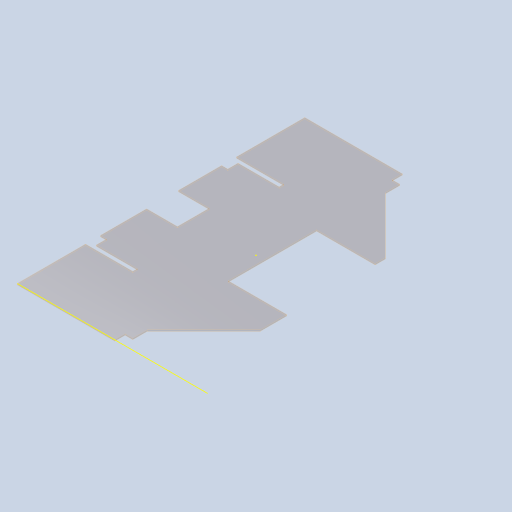
# Autodesk Inventor part: DB1-015
Saved by Autodesk Inventor 2023.4 (Build 274418000, 418)
## iProperties
Created: 2025-02-19
Part Number: DB1-015
Material: Polycarbonate, Smoke
Document SubType Name: Sheet Metal
Designer: AIM
Density: 1.2 g/cm^3
Sheet Metal Rule: Default
Appearance: Polycarbonate - Smoked
Author: AIM
Autodesk Inventor part; units mm, degrees
ref_plane "YZ Plane" through (0, 0, 0) normal (1, 0, 0) x (0, 1, 0)
ref_plane "XZ Plane" through (0, 0, 0) normal (0, 1, 0) x (-1, 0, 0)
ref_plane "XY Plane" through (0, 0, 0) normal (0, 0, 1) x (1, 0, 0)
sketch "Sketch1" plane through (0, 0, 0) normal (0, 1, 0) x (-1, 0, 0)
  line L0 (234.95, 355.6) -> (-234.95, 355.6)
  line L1 (-234.95, 355.6) -> (-234.95, -355.6)
  line L2 (-234.95, -355.6) -> (234.95, -355.6)
  line L3 (234.95, -355.6) -> (234.95, 355.6)
  line L4 (234.95, 355.6) -> (-234.95, -355.6) construction
  line L5 (-234.95, 355.6) -> (234.95, -355.6) construction
  point P0 (0, 0)
  dimension "d0" = 469.9
  dimension "d1" = 711.2
  measures "d0" distance of L2.end L1.end
  measures "d1" distance of L1.end L0.end
extrude "Plate1" add sketch "Sketch1" along normal blind 3.048
sketch "Sketch3" plane through (0, 3.048, 0) normal (0, 1, 0) x (1, 0, 0)
  line L0 (234.95, -355.6) -> (-234.95, -355.6) projected
  point P0 (0, 0)
sketch "Sketch4" plane through (0, 0, 0) normal (0, -1, 0) x (1, 0, 0)
  line L0 (-234.95, 355.6) -> (234.95, 355.6) projected
  line L1 (-234.95, -355.6) -> (-234.95, 355.6) projected
  line L2 (234.95, -355.6) -> (-234.95, -355.6) projected
  line L3 (234.95, 355.6) -> (234.95, -355.6) projected
  line L4 (-234.95, 355.6) -> (234.95, 355.6) projected
  line L5 (25.4, 355.6) -> (25.4, 294.64)
  line L6 (165.1, 101.6) -> (234.95, 101.6)
  line L7 (234.95, 355.6) -> (234.95, -355.6) projected
  line L8 (25.4, 294.64) -> (165.1, 154.94)
  line L9 (25.4, 294.64) -> (222.9656, 294.64) construction
  line L10 (165.1, 154.94) -> (165.1, 101.6)
  line L11 (234.95, 0) -> (-234.95, 0)
  line L12 (-234.95, -355.6) -> (-234.95, 355.6) projected
  line L13 (25.4, -355.6) -> (25.4, -294.64)
  line L14 (165.1, -127) -> (234.95, -127)
  line L15 (25.4, -294.64) -> (165.1, -154.94)
  line L16 (25.4, -294.64) -> (222.9656, -294.64) construction
  line L17 (165.1, -154.94) -> (165.1, -127)
  line L18 (-234.95, 184.15) -> (-120.65, 184.15)
  line L19 (-120.65, 184.15) -> (-120.65, 177.8)
  line L20 (-120.65, 177.8) -> (-222.25, 177.8)
  line L21 (-222.25, 177.8) -> (-222.25, 152.4)
  line L22 (-222.25, 152.4) -> (-234.95, 152.4)
  line L23 (-234.95, 149.86) -> (-219.71, 149.86)
  line L24 (-219.71, 149.86) -> (-219.71, 175.26)
  line L25 (-219.71, 175.26) -> (-118.11, 175.26)
  line L26 (-118.11, 175.26) -> (-118.11, 186.69)
  line L27 (-118.11, 186.69) -> (-234.95, 186.69)
  line L28 (165.1, -129.54) -> (20.32, -129.54)
  line L29 (20.32, -129.54) -> (20.32, 88.9)
  line L30 (20.32, 88.9) -> (165.1, 88.9)
  line L31 (165.1, 101.6) -> (165.1, 88.9)
  line L32 (-234.95, -184.15) -> (-120.65, -184.15)
  line L33 (-120.65, -184.15) -> (-120.65, -177.8)
  line L34 (-120.65, -177.8) -> (-222.25, -177.8)
  line L35 (-222.25, -177.8) -> (-222.25, -152.4)
  line L36 (-222.25, -152.4) -> (-234.95, -152.4)
  line L37 (-234.95, -149.86) -> (-219.71, -149.86)
  line L38 (-219.71, -149.86) -> (-219.71, -175.26)
  line L39 (-219.71, -175.26) -> (-118.11, -175.26)
  line L40 (-118.11, -175.26) -> (-118.11, -186.69)
  line L41 (-118.11, -186.69) -> (-234.95, -186.69)
  line L42 (-158.75, 35.56) -> (-158.75, -43.18)
  line L43 (-158.75, -43.18) -> (-234.95, -43.18)
  line L44 (-158.75, 35.56) -> (-234.95, 35.56)
  line L45 (25.4, 330.2) -> (6.35, 330.2)
  line L46 (6.35, 330.2) -> (6.35, 355.6)
  line L47 (25.4, -330.2) -> (6.35, -330.2)
  line L48 (6.35, -330.2) -> (6.35, -355.6)
  line L49 (234.95, -355.6) -> (-234.95, -355.6) projected
  point P0 (0, 0)
  dimension "d3" = 209.55
  dimension "d4" = 254
  dimension "d5" = 45
  dimension "d6" = 60.96
  dimension "d9" = 69.85
  dimension "d12" = 45
  dimension "d13" = 209.55
  dimension "d14" = 228.6
  dimension "d15" = 69.85
  dimension "d16" = 60.96
  dimension "d17" = 171.45
  dimension "d18" = 114.3
  dimension "d19" = 6.35
  dimension "d21" = 101.6
  dimension "d22" = 25.4
  dimension "d23" = 2.54
  dimension "d26" = 144.78
  dimension "d31" = 12.7
  dimension "d32" = 114.3
  dimension "d33" = 171.45
  dimension "d34" = 6.35
  dimension "d35" = 101.6
  dimension "d36" = 25.4
  dimension "d37" = 2.54
  dimension "d38" = 76.2
  dimension "d39" = 35.56
  dimension "d40" = 43.18
  dimension "d41" = 2.54
  dimension "d42" = 25.4
  dimension "d43" = 19.05
  dimension "d44" = 25.4
  dimension "d45" = 19.05
  constraints: 84 end point, 14 horizontal, 11 point on line, 8 vertical, 4 perpendicular, 2 midpoint, 1 equal length, 1 vertical alignment, 19 other
  measures "d3" distance between parallel lines of L3 L5
  measures "d4" distance between parallel lines of L0 L6
  measures "d5" angle of L8 L9
  measures "d6" distance from line of L5.end L0
  measures "d9" distance between parallel lines of L3 L10
  measures "d12" angle of L15 L16
  measures "d13" distance between parallel lines of L3 L13
  measures "d14" distance between parallel lines of L2 L14
  measures "d15" distance between parallel lines of L3 L17
  measures "d16" distance from line of L13.end L2
  measures "d17" distance between parallel lines of L0 L18
  measures "d18" distance of L18.start L18.end
  measures "d19" distance of L18.end L19.end
  measures "d21" distance of L19.end L20.end
  measures "d22" distance of L20.end L21.end
  measures "d23" distance between parallel lines of L20 L25
  measures "d26" distance of L28.start L28.end
  measures "d31" distance of L6.start L30.end
  measures "d32" distance of L32.start L32.end
  measures "d33" distance between parallel lines of L2 L32
  measures "d34" distance of L32.end L33.end
  measures "d35" distance of L33.end L34.end
  measures "d36" distance of L34.end L35.end
  measures "d37" distance between parallel lines of L34 L39
  measures "d38" distance between parallel lines of L1 L42
  measures "d39" distance from line of point (-234.95, 0) L44
  measures "d40" distance from line of point (-234.95, 0) L43
  measures "d41" distance of L14.start L28.start
  measures "d42" distance of L45.end L46.end
  measures "d43" distance of L45.start L45.end
  measures "d44" distance of L47.end L48.end
  measures "d45" distance of L47.start L47.end
extrude "Cut1" cut sketch "Sketch4" against normal blind 3.048 contours L27 L26 L25 L24 L23 L1 L22 L21 L20 L19 L18 | L0 L3 L6 L10 L8 L5 | L18 L19 L20 L21 L22 L1 | L3 L11 L29 L30 L31 L6 | L3 L14 L17 L28 L29 L11 | L44 L42 L11 L1 | L3 L2 L13 L15 L17 L14 | L11 L42 L43 L1 | L37 L38 L39 L40 L41 L1 L32 L33 L34 L35 L36 | L36 L35 L34 L33 L32 L1
sketch "Sketch5" plane through (0, 0, 0) normal (0, -1, 0) x (1, 0, 0)
  line L0 (25.4, 355.6) -> (25.4, 294.64) projected
  line L1 (25.4, 294.64) -> (165.1, 154.94) projected
  line L2 (165.1, 154.94) -> (165.1, 88.9) projected
  line L3 (165.1, 88.9) -> (20.32, 88.9) projected
  line L4 (20.32, 88.9) -> (20.32, -129.54) projected
  line L5 (20.32, -129.54) -> (165.1, -129.54) projected
  line L6 (165.1, -129.54) -> (165.1, -154.94) projected
  line L7 (165.1, -154.94) -> (25.4, -294.64) projected
  line L8 (25.4, -294.64) -> (25.4, -355.6) projected
  line L9 (25.4, -355.6) -> (-234.95, -355.6) projected
  line L10 (-234.95, -355.6) -> (-234.95, -186.69) projected
  line L11 (-234.95, -186.69) -> (-118.11, -186.69) projected
  line L12 (-118.11, -186.69) -> (-118.11, -175.26) projected
  line L13 (-118.11, -175.26) -> (-219.71, -175.26) projected
  line L14 (-219.71, -175.26) -> (-219.71, -149.86) projected
  line L15 (-219.71, -149.86) -> (-234.95, -149.86) projected
  line L16 (-234.95, -149.86) -> (-234.95, -43.18) projected
  line L17 (-234.95, -43.18) -> (-158.75, -43.18) projected
  line L18 (-158.75, -43.18) -> (-158.75, 35.56) projected
  line L19 (-158.75, 35.56) -> (-234.95, 35.56) projected
  line L20 (-234.95, 35.56) -> (-234.95, 149.86) projected
  line L21 (-234.95, 149.86) -> (-219.71, 149.86) projected
  line L22 (-219.71, 149.86) -> (-219.71, 175.26) projected
  line L23 (-219.71, 175.26) -> (-118.11, 175.26) projected
  line L24 (-118.11, 175.26) -> (-118.11, 186.69) projected
  line L25 (-118.11, 186.69) -> (-234.95, 186.69) projected
  line L26 (-234.95, 186.69) -> (-234.95, 355.6) projected
  line L27 (-234.95, 355.6) -> (25.4, 355.6) projected
  line L28 (25.4, -355.6) -> (-234.95, -355.6) projected
  line L29 (25.4, -355.6) -> (6.35, -355.6)
  line L30 (6.35, -355.6) -> (6.35, -330.2)
  line L31 (6.35, -330.2) -> (25.4, -330.2)
  line L32 (25.4, -330.2) -> (25.4, -355.6)
  line L33 (-234.95, 355.6) -> (25.4, 355.6) projected
  line L34 (25.4, 355.6) -> (6.35, 355.6)
  line L35 (6.35, 355.6) -> (6.35, 330.2)
  line L36 (6.35, 330.2) -> (25.4, 330.2)
  line L37 (25.4, 330.2) -> (25.4, 355.6)
  point P0 (0, 0)
  dimension "d46" = 19.05
  dimension "d47" = 25.4
  dimension "d48" = 19.05
  dimension "d49" = 25.4
  constraints: 16 end point, 4 parallel, 2 horizontal, 2 perpendicular
  measures "d46" distance of L30.end L31.end
  measures "d47" distance of L29.end L30.end
  measures "d48" distance of L36.end L35.end
  measures "d49" distance of L35.end L34.end
extrude "Cut2" cut sketch "Sketch5" against normal blind 3.048 contours L0 L36 L35 L27 | L8 L9 L30 L31
equation "\"d10\" = Thickness"
equation "\"d2\" = Thickness"
equation "\"BendRadius\" = Thickness"
equation "\"BendReliefWidth\" = Thickness"
equation "\"BendReliefDepth\" = 0.5 * Thickness"
equation "\"CornerReliefSize\" = 4 * Thickness"
equation "\"MinimumRemnant\" = 2 * Thickness"
equation "\"TransitionRadius\" = BendRadius"
equation "\"JacobiRadiusSize\" = BendRadius"
equation "\"GapSize\" = Thickness"
equation "\"Thickness\" = 3.048"
body "Solid1"
